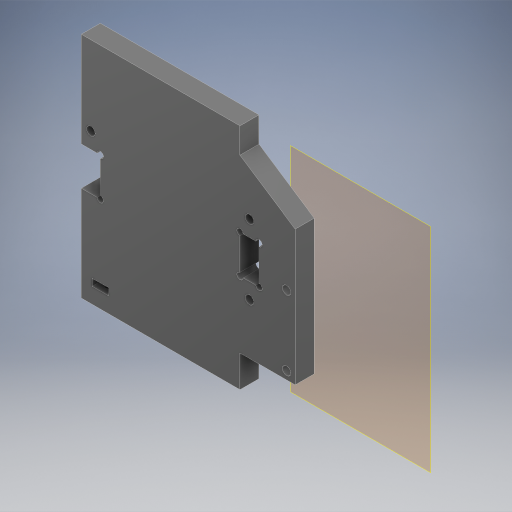
# Autodesk Inventor part: side of head
Saved by Autodesk Inventor 2024 (Build 280153000, 153)
## iProperties
Created: 2024-09-04
Part Number: side of head
Material: PMMA 플라스틱
Document SubType Name: Modeling
Designer: msi
Density: 1.188 g/cm^3
Appearance: 매끄러움 - 검은색
Mass: 30.2077 g
Surface Area: 109.051 cm^2
Volume: 25.4274 cm^3
Author: msi
Autodesk Inventor part; units mm, degrees
ref_plane "YZ Plane" through (0, 0, 0) normal (1, 0, 0) x (0, 1, 0)
ref_plane "XZ Plane" through (0, 0, 0) normal (0, 1, 0) x (-1, 0, 0)
ref_plane "XY Plane" through (0, 0, 0) normal (0, 0, 1) x (1, 0, 0)
ref_plane "작업 평면1" through (0, 0, 0) normal (0, 0, 1) x (1, 0, 0)
sketch "스케치1" plane through (0, 0, 0) normal (0, 0, 1) x (1, 0, 0)
  arc A0 (20.1, 4.5766) -> (19.5808, 6.2636) centre (17.1, 4.5766) ccw projected
  line L0 (19.5808, 6.2636) -> (15.5953, 12.1246) projected
  arc A1 (15.5953, 12.1246) -> (13.9414, 13) centre (13.9414, 11) ccw projected
  line L1 (13, 13) -> (13.9414, 13) projected
  arc A2 (14.5, 11.5) -> (13, 13) centre (13, 11.5) ccw projected
  line L2 (14.5, -41.5) -> (14.5, 11.5) projected
  arc A3 (13.5, -42.5) -> (14.5, -41.5) centre (13.5, -41.5) ccw projected
  line L3 (-13.5, -42.5) -> (13.5, -42.5) projected
  arc A4 (-14.5, -41.5) -> (-13.5, -42.5) centre (-13.5, -41.5) ccw projected
  line L4 (-14.5, 11.5) -> (-14.5, -41.5) projected
  arc A5 (-13, 13) -> (-14.5, 11.5) centre (-13, 11.5) ccw projected
  line L5 (-13.9414, 13) -> (-13, 13) projected
  arc A6 (-13.9414, 13) -> (-15.5953, 12.1246) centre (-13.9414, 11) ccw projected
  line L6 (-15.5953, 12.1246) -> (-19.5808, 6.2636) projected
  arc A7 (-19.5808, 6.2636) -> (-20.1, 4.5766) centre (-17.1, 4.5766) ccw projected
  line L7 (-20.1, 4.5766) -> (-20.1, -39.6766) projected
  arc A8 (-20.1, -39.6766) -> (-19.5808, -41.3636) centre (-17.1, -39.6766) ccw projected
  line L8 (-19.5808, -41.3636) -> (-15.8929, -46.7869) projected
  arc A9 (-15.8929, -46.7869) -> (-13.4121, -48.1) centre (-13.4121, -45.1) ccw projected
  line L9 (-13.4121, -48.1) -> (13.4121, -48.1) projected
  arc A10 (13.4121, -48.1) -> (15.8929, -46.7869) centre (13.4121, -45.1) ccw projected
  line L10 (15.8929, -46.7869) -> (19.5808, -41.3636) projected
  arc A11 (19.5808, -41.3636) -> (20.1, -39.6766) centre (17.1, -39.6766) ccw projected
  line L11 (20.1, -39.6766) -> (20.1, 4.5766) projected
  circle A12 centre (-17.3, 4) radius 1.35 projected
  circle A13 centre (-17.3, -18) radius 1.35 projected
  circle A14 centre (-11, -45.3) radius 1.35 projected
  circle A15 centre (17.3, 4) radius 1.35 projected
  circle A16 centre (17.3, -18) radius 1.35 projected
  circle A17 centre (11, -45.3) radius 1.35 projected
  circle A18 centre (-17.3, -40) radius 1.35 projected
  circle A19 centre (17.3, -40) radius 1.35 projected
  arc A20 (-14.6, -41.5) -> (-13.5, -42.6) centre (-13.5, -41.5) ccw
  line L12 (-13.5, -42.6) -> (13.5, -42.6)
  arc A21 (13.5, -42.6) -> (14.6, -41.5) centre (13.5, -41.5) ccw
  line L13 (14.6, -41.5) -> (14.6, 11.5)
  arc A22 (14.6, 11.5) -> (12.2254, 12.9) centre (13, 11.5) ccw
  line L14 (12.2254, 12.9) -> (13.9414, 12.9)
  arc A23 (15.5126, 12.0684) -> (13.9414, 12.9) centre (13.9414, 11) ccw
  line L15 (15.5126, 12.0684) -> (19.4981, 6.2073)
  arc A24 (20, 4.5766) -> (19.4981, 6.2073) centre (17.1, 4.5766) ccw
  line L16 (20, 4.5766) -> (20, -39.6766)
  arc A25 (19.4981, -41.3073) -> (20, -39.6766) centre (17.1, -39.6766) ccw
  line L17 (19.4981, -41.3073) -> (15.8102, -46.7307)
  arc A26 (13.4121, -48) -> (15.8102, -46.7307) centre (13.4121, -45.1) ccw
  line L18 (13.4121, -48) -> (-13.4121, -48)
  arc A27 (-15.8102, -46.7307) -> (-13.4121, -48) centre (-13.4121, -45.1) ccw
  line L19 (-15.8102, -46.7307) -> (-18.6871, -42.5)
  line L20 (-19.4981, 6.2073) -> (-15.5126, 12.0684)
  arc A28 (-13.9414, 12.9) -> (-15.5126, 12.0684) centre (-13.9414, 11) ccw
  line L21 (-13.9414, 12.9) -> (-12.2254, 12.9)
  arc A29 (-12.2254, 12.9) -> (-14.6, 11.5) centre (-13, 11.5) ccw
  line L22 (-14.6, 11.5) -> (-14.6, -41.5)
  line L23 (-14.6, 11.5) -> (-20, 11.5)
  line L24 (-20, -42.5) -> (-14.6, -42.5)
  line L25 (-14.6, -42.5) -> (-14.6, 11.5)
  line L26 (-20, 11.5) -> (-32, 11.5)
  line L27 (-32, -42.5) -> (-20, -42.5)
  circle A30 centre (-17.3, 4) radius 1.35
  circle A31 centre (-17.3, -18) radius 1.35
  circle A32 centre (-17.3, -40) radius 1.35
  line L28 (-32, -9.5) -> (-26, -9.5)
  line L29 (-26, -9.5) -> (-26, -21.5)
  line L30 (-26, -21.5) -> (-32, -21.5)
  line L31 (-32, 11.5) -> (-32, -9.5)
  line L32 (-32, -21.5) -> (-32, -42.5)
  circle A33 centre (-29, -4.5) radius 1.35
  circle A34 centre (-29, -26.5) radius 1.35
  point P0 (0, 0)
  dimension "d0" = 0.1
  dimension "d2" = 2.7
  dimension "d3" = 2.7
  dimension "d4" = 2.7
  dimension "d5" = 12
  dimension "d6" = 2.7
  dimension "d7" = 2.7
  constraints: 42 end point, 20 point on circle, 15 centre point, 3 coincident, 3 horizontal, 3 parallel, 3 perpendicular, 1 point on line, 18 other
  measures "d0" distance between parallel lines of L4 L22
  measures "d2" diameter of A30
  measures "d3" diameter of A31
  measures "d4" diameter of A32
  measures "d5" distance of L28.end L29.end
  measures "d6" diameter of A33
  measures "d7" diameter of A34
extrude "돌출1" add sketch "스케치1" along normal blind 6 contours L24 L27 L32 L30 L29 L28 L31 L26 L23 L6 A7 L7 A8 L8 | L8 A8 L7 A7 L6 L23 L22 L25 L24
sketch "스케치2" plane through (-32, -42.5, 0) normal (-1, 0, 0) x (0, 0, 1)
  line L0 (0, 62) -> (6, 62)
  line L1 (6, 62) -> (6, -10)
  line L2 (6, -10) -> (0, -10)
  line L3 (0, -10) -> (0, 62)
  point P0 (0, 42.5)
  dimension "d10" = 6
  dimension "d11" = 72
  constraints: 8 end point, 2 parallel, 1 horizontal, 1 perpendicular
  measures "d10" distance of L1.end L2.end
  measures "d11" distance of L0.end L1.end
extrude "돌출2" add sketch "스케치2" along normal blind 50
sketch "스케치3" plane through (0, 0, 6) normal (0, 0, 1) x (1, 0, 0)
  line L0 (-32, -42.5) -> (-14.6, -42.5) projected
  line L1 (-14.6, -42.5) -> (-14.6, 11.5) projected
  line L2 (-14.6, 11.5) -> (-32, 11.5) projected
  line L3 (-32, 11.5) -> (-32, 19.5) projected
  line L4 (-32, 19.5) -> (-82, 19.5) projected
  line L5 (-82, -52.5) -> (-82, 19.5) projected
  line L6 (-32, -52.5) -> (-82, -52.5) projected
  line L7 (-32, -52.5) -> (-32, -42.5) projected
  line L8 (-32, -21.5) -> (-32, -9.5) projected
  line L9 (-32, -9.5) -> (-26, -9.5) projected
  line L10 (-26, -9.5) -> (-26, -21.5) projected
  line L11 (-26, -21.5) -> (-32, -21.5) projected
  circle A0 centre (-17.3, -18) radius 1.35 projected
  circle A1 centre (-17.3, 4) radius 1.35 projected
  circle A2 centre (-17.3, -40) radius 1.35 projected
  circle A3 centre (-29, -26.5) radius 1.35 projected
  circle A4 centre (-29, -4.5) radius 1.35 projected
  line L12 (-14.6, 0) -> (-32, 11.5)
  line L13 (-32, 11.5) -> (-14.6, 11.5)
  point P0 (0, 0)
  constraints: 4 end point, 1 horizontal, 1 point on line
extrude "돌출3" cut sketch "스케치3" against normal blind 50 contours L12 L2 L1
sketch "스케치5" plane through (-82, -42.5, 0) normal (-1, 0, 0) x (0, 0, 1)
  line L0 (-2.9941, 20.5626) -> (2.9941, 31.4374) construction
  line L1 (2.9941, 20.5626) -> (-2.9941, 31.4374) construction
  line L2 (0, 20) -> (0, 32)
  line L3 (6, 32) -> (6, 20)
  line L4 (6, 20) -> (0, 32) construction
  line L5 (0, 20) -> (6, 32) construction
  line L6 (6.025, 19.95) -> (-0.025, 19.95)
  line L7 (-0.025, 19.95) -> (-0.025, 32.05)
  line L8 (-0.025, 32.05) -> (6.025, 32.05)
  line L9 (6.025, 32.05) -> (6.025, 19.95)
  line L10 (6.025, 19.95) -> (-0.025, 32.05) construction
  line L11 (-0.025, 19.95) -> (6.025, 32.05) construction
  point P0 (0, 42.5)
  point P1 (0, 26)
  point P2 (3, 26)
  dimension "d16" = 6
  dimension "d17" = 12
  dimension "d18" = 12.1
  constraints: 24 end point, 5 midpoint, 3 parallel, 1 horizontal, 1 perpendicular, 1 point on line
  measures "d16" distance of L2.end L3.start
  measures "d17" distance of L2.start L2.end
  measures "d18" distance of L6.end L7.end
extrude "돌출4" cut sketch "스케치5" against normal blind 6
sketch "스케치6" plane through (0, 0, 6) normal (0, 0, 1) x (1, 0, 0)
  line L0 (-76, -10.45) -> (-76, -22.55) projected
  line L1 (-82, -10.45) -> (-76, -10.45) projected
  line L2 (-76, -22.55) -> (-82, -22.55) projected
  circle A0 centre (-79, -5.45) radius 1.35
  point P0 (0, 0)
  dimension "d21" = 2.7
  constraints: 1 centre point
  measures "d21" diameter of A0
extrude "돌출5" cut sketch "스케치6" against normal blind 6
sketch "스케치7" plane through (-32, -52.5, 0) normal (0, -1, 0) x (1, 0, 0)
  line L0 (0, 0) -> (0, 6) projected
  line L1 (0, 6) -> (-50, 6) projected
  line L2 (-50, 0) -> (-50, 6) projected
  line L3 (0, 0) -> (-50, 0) projected
  circle A0 centre (-44, 3) radius 1.35
  point P0 (32, 0)
  dimension "d24" = 2.7
  constraints: 1 centre point
  measures "d24" diameter of A0
extrude "돌출6" cut sketch "스케치7" against normal blind 20 contours A0
sketch "스케치8" plane through (0, 0, 6) normal (0, 0, 1) x (1, 0, 0)
  circle A0 centre (-79, -5.45) radius 1.35 projected
  line L0 (-76, -22.55) -> (-82, -22.55) projected
  line L1 (-82, -52.5) -> (-82, -22.55) projected
  line L2 (-32, -52.5) -> (-82, -52.5) projected
  line L3 (-32, -52.5) -> (-32, -42.5) projected
  line L4 (-32, -42.5) -> (-14.6, -42.5) projected
  line L5 (-14.6, -42.5) -> (-14.6, 0) projected
  line L6 (-14.6, 0) -> (-32, 11.5) projected
  line L7 (-32, 11.5) -> (-32, 19.5) projected
  line L8 (-32, 19.5) -> (-82, 19.5) projected
  line L9 (-82, -10.45) -> (-82, 19.5) projected
  line L10 (-82, -10.45) -> (-76, -10.45) projected
  line L11 (-76, -10.45) -> (-76, -22.55) projected
  line L12 (-32, -21.5) -> (-32, -9.5) projected
  line L13 (-32, -9.5) -> (-26, -9.5) projected
  line L14 (-26, -9.5) -> (-26, -21.5) projected
  line L15 (-26, -21.5) -> (-32, -21.5) projected
  circle A1 centre (-17.3, -18) radius 1.35 projected
  circle A2 centre (-17.3, -40) radius 1.35 projected
  circle A3 centre (-29, -26.5) radius 1.35 projected
  circle A4 centre (-29, -4.5) radius 1.35 projected
  line L16 (-73.4, -45.4) -> (-78.6, -45.4)
  line L17 (-78.6, -45.4) -> (-78.6, -47.6)
  line L18 (-78.6, -47.6) -> (-73.4, -47.6)
  line L19 (-73.4, -47.6) -> (-73.4, -45.4)
  line L20 (-73.4, -45.4) -> (-78.6, -47.6) construction
  line L21 (-78.6, -45.4) -> (-73.4, -47.6) construction
  point P0 (0, 0)
  point P1 (-76, -46.5)
  dimension "d27" = 5.2
  dimension "d28" = 2.2
  constraints: 12 end point, 2 midpoint, 2 parallel, 1 horizontal, 1 perpendicular
  measures "d27" distance of L18.end L17.end
  measures "d28" distance of L17.end L16.end
extrude "돌출7" cut sketch "스케치8" against normal blind 20 contours L19 L18 L17 L16
sketch "스케치9" plane through (0, 0, 6) normal (0, 0, 1) x (1, 0, 0)
  line L0 (-76, -10.45) -> (-76, -22.55) projected
  line L1 (-82, -10.45) -> (-76, -10.45) projected
  line L2 (-76, -22.55) -> (-82, -22.55) projected
  line L3 (-32, -21.5) -> (-32, -9.5) projected
  line L4 (-32, -9.5) -> (-26, -9.5) projected
  line L5 (-26, -9.5) -> (-26, -21.5) projected
  line L6 (-26, -21.5) -> (-32, -21.5) projected
  circle A0 centre (-76, -10.45) radius 1
  circle A1 centre (-76, -22.55) radius 1
  circle A2 centre (-32, -9.5) radius 1
  circle A3 centre (-26, -9.5) radius 1
  circle A4 centre (-26, -21.5) radius 1
  circle A5 centre (-32, -21.5) radius 1
  point P0 (0, 0)
  dimension "d31" = 2
  dimension "d32" = 2
  dimension "d33" = 2
  dimension "d34" = 2
  dimension "d35" = 2
  dimension "d36" = 2
  constraints: 6 centre point, 6 coincident
  measures "d31" diameter of A0
  measures "d32" diameter of A1
  measures "d33" diameter of A2
  measures "d34" diameter of A3
  measures "d35" diameter of A4
  measures "d36" diameter of A5
extrude "돌출8" cut sketch "스케치9" against normal blind 10 contours L1 A0 L0 | L0 A0 L1 | A1 L2 L0 | L0 L2 A1 | L6 A5 L3 | L3 A5 L6 | A2 L4 L3 | L3 L4 A2 | A4 L5 L6 | L6 L5 A4 | A3 L5 L4 | L4 L5 A3
